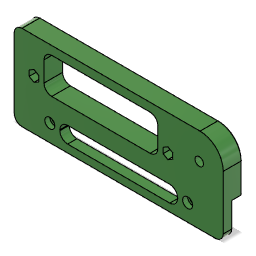
RFVplotter-PSUMountingBracketRight-v1_0 (Autodesk Fusion 360 design; units mm, degrees)
Autodesk Fusion 360 part; units mm, degrees
sketch "Sketch1" plane through (0, 0, 0) normal (0, 0, 1) x (1, 0, 0)
  line L0 (67.5, 27.5) -> (-67.5, 27.5)
  line L1 (-67.5, 27.5) -> (-67.5, -27.5)
  line L2 (-67.5, -27.5) -> (67.5, -27.5)
  line L3 (67.5, -27.5) -> (67.5, 27.5)
  line L4 (67.5, 27.5) -> (-67.5, -27.5) construction
  line L5 (-67.5, 27.5) -> (67.5, -27.5) construction
  dimension "d1" = 55
  dimension "d2" = 135
  constraint horizontal L0
  constraint perpendicular L0 L1
  constraint parallel L0 L2
  constraint parallel L1 L3
  constraint coincident L4 origin
  constraint coincident L5 origin
  measures "d1" distance of L0.end L1.end
  measures "d2" distance of L1.end L2.end
extrude "Extrude1" add sketch "Sketch1" along normal blind 6
sketch "Sketch3" plane through (0, 0, 0) normal (0, 0, -1) x (-1, 0, 0)
  line L0 (-67.5, 27.5) -> (-67.5, -27.5)
  line L1 (-67.5, -27.5) -> (67.5, -27.5)
  line L2 (67.5, -27.5) -> (67.5, 27.5)
  line L3 (67.5, 27.5) -> (-67.5, 27.5)
  line L4 (-67.5, -7) -> (67.5, -7)
  line L5 (67.5, -7) -> (67.5, 27.5)
  line L6 (67.5, 27.5) -> (-67.5, 27.5)
  line L7 (-67.5, 27.5) -> (-67.5, -7)
  line L8 (-67.5, -7) -> (67.5, 27.5) construction
  line L9 (67.5, -7) -> (-67.5, 27.5) construction
  point P0 (0, 10.25)
  dimension "d14" = 34.5
  dimension "d30" = 20.5
  constraint horizontal L4
  constraint perpendicular L4 L5
  constraint parallel L4 L6
  constraint parallel L5 L7
  constraint coincident L8 P0
  constraint coincident L9 P0
  constraint collinear L2 L5
  constraint collinear L3 L6
  constraint collinear L0 L7
  measures "d14" distance of L4.end L2.end
  measures "d30" distance of L1 L4
extrude "Extrude2" add sketch "Sketch3" along normal blind 6 contours L0 L2 L3 L4 L5 L6 L7
sketch "Sketch2" plane through (0, 0, 6) normal (0, 0, 1) x (1, 0, 0)
  line L0 (67.5, -27.5) -> (67.5, 27.5)
  line L1 (67.5, 27.5) -> (-67.5, 27.5)
  line L2 (-67.5, 27.5) -> (-67.5, -27.5)
  line L3 (-67.5, -27.5) -> (67.5, -27.5)
  line L4 (67.5, -7) -> (-67.5, -7)
  point P0 (-44.5, -16.5)
  point P1 (44.5, -16.5)
  dimension "d7" = 23
  dimension "d47" = 9.5
  dimension "d48" = 9.5
  dimension "d49" = 89
  measures "d7" distance of L0 P1
  measures "d47" distance of P1 L4
  measures "d48" distance of P0 L4
  measures "d49" horizontal distance of P0 P1
hole "Hole1" at (-44.5, -16.5, 6) at (44.5, -16.5, 6) direction (0, 0, -1) diameter 3.5 end through all counterbore diameter 6.5 counterbore depth 3.25
sketch "Sketch4" plane through (0, 0, -6) normal (0, 0, -1) x (-1, 0, 0)
  line L0 (-67.5, 27.5) -> (-67.5, -7)
  line L1 (-67.5, -7) -> (67.5, -7)
  line L2 (67.5, -7) -> (67.5, 27.5)
  line L3 (67.5, 27.5) -> (-67.5, 27.5)
  line L4 (-67.5, 4.75) -> (67.5, 4.75) construction
  point P0 (54.75, 4.75)
  point P1 (-31.75, 4.75)
  dimension "d19" = 12.75
  dimension "d20" = 86.5
  dimension "d31" = 11.75
  constraint coincident L0 L4.start
  constraint coincident L2 L4.end
  constraint perpendicular L2 L4
  constraint coincident L4 P0
  constraint coincident L4 P1
  measures "d19" distance of L2 P0
  measures "d20" distance of P0 P1
  measures "d31" distance of L1 L4
hole "Hole2" at (31.75, 4.75, -6) at (-54.75, 4.75, -6) direction (0, 0, 1) diameter 3.5 end through all
sketch "Sketch5" plane through (0, 0, 6) normal (0, 0, 1) x (1, 0, 0)
  circle A0 centre (31.75, 4.75) radius 1.75
  circle A1 centre (-54.75, 4.75) radius 1.75
  circle A2 centre (-44.5, -16.5) radius 3.25
  circle A3 centre (44.5, -16.5) radius 3.25
  line L0 (67.5, -27.5) -> (67.5, 27.5)
  line L1 (67.5, 27.5) -> (-67.5, 27.5)
  line L2 (-67.5, 27.5) -> (-67.5, -27.5)
  line L3 (-67.5, -27.5) -> (67.5, -27.5)
  line L4 (-51.65, 6.5398) -> (-54.75, 8.3296)
  line L5 (-54.75, 8.3296) -> (-57.85, 6.5398)
  line L6 (-57.85, 6.5398) -> (-57.85, 2.9602)
  line L7 (-57.85, 2.9602) -> (-54.75, 1.1704)
  line L8 (-54.75, 1.1704) -> (-51.65, 2.9602)
  line L9 (-51.65, 2.9602) -> (-51.65, 6.5398)
  line L10 (34.85, 2.9602) -> (34.85, 6.5398)
  line L11 (34.85, 6.5398) -> (31.75, 8.3296)
  line L12 (31.75, 8.3296) -> (28.65, 6.5398)
  line L13 (28.65, 6.5398) -> (28.65, 2.9602)
  line L14 (28.65, 2.9602) -> (31.75, 1.1704)
  line L15 (31.75, 1.1704) -> (34.85, 2.9602)
  point P0 (-54.75, 4.75)
  point P1 (31.75, 4.75)
  dimension "d24" = 6.2
  dimension "d25" = 6.2
  constraint coincident P0 A1.centre
  constraint vertical L9
  constraint coincident A0.centre P1
  constraint vertical L10
  measures "d24" distance of L6 L9
  measures "d25" distance of L10 L13
extrude "Extrude3" cut sketch "Sketch5" against normal blind 6 contours L4 L5 L6 L7 L8 L9 | L10 L11 L12 L13 L14 L15
sketch "Sketch6" plane through (0, 0, -6) normal (0, 0, -1) x (-1, 0, 0)
  circle A0 centre (-31.75, 4.75) radius 1.75
  circle A1 centre (54.75, 4.75) radius 1.75
  line L0 (-67.5, 27.5) -> (-67.5, -7)
  line L1 (-67.5, -7) -> (67.5, -7)
  line L2 (67.5, -7) -> (67.5, 27.5)
  line L3 (67.5, 27.5) -> (-67.5, 27.5)
  line L4 (59.5, -7) -> (-36.5, -7) construction
  line L5 (-36.5, -7) -> (-36.5, 28) construction
  line L6 (-36.5, 28) -> (59.5, 28) construction
  line L7 (59.5, 28) -> (59.5, -7) construction
  line L8 (59.5, -7) -> (-36.5, 28) construction
  line L9 (-36.5, -7) -> (59.5, 28) construction
  line L10 (11.5, 50.5144) -> (11.5, -41.0982) construction
  line L11 (-52, 27.5) -> (-52, -7) construction
  line L12 (-36.5, 10.25) -> (-67.5, 10.25) construction
  point P0 (11.5, 10.5)
  point P1 (-52, 10.25)
  dimension "d28" = 35
  dimension "d29" = 96
  constraint horizontal L4
  constraint perpendicular L4 L5
  constraint parallel L4 L6
  constraint parallel L5 L7
  constraint coincident L8 P0
  constraint coincident L9 P0
  constraint collinear L1 L4
  constraint perpendicular L4 L10
  constraint symmetric A0.centre A1.centre L10
  constraint coincident P0 L10
  constraint coincident L3 L11.start
  constraint coincident L1 L11.end
  constraint perpendicular L1 L11
  constraint coincident L5 L12.start
  constraint coincident L0 L12.end
  constraint perpendicular L0 L12
  constraint symmetric L1 L3 L12
  constraint coincident L11 P1
  constraint coincident L12 P1
  measures "d28" distance of L4.start L6.end
  measures "d29" distance of L5.end L6.end
hole "Hole3" at (52, 10.25, -6) direction (0, 0, 1) diameter 5.5 end through all
fillet "Fillet1" radius 5 2 edges at (67.5, -27.5, 3) (-67.5, -27.5, 3)
fillet "Fillet1" radius 5 1 edges at (-67.5, 27.5, 0)
fillet "Fillet3" radius 15 1 edges at (67.5, 27.5, 0)
fillet "Fillet4" radius 1 1 edges at (0, -7, -6)
fillet "Fillet5" radius 0.5 14 edges at (-67.5, -14.75, 0) (-66.0355, -26.0355, 0) (0, -27.5, 0) (66.0355, -26.0355, 0) (67.5, -14.75, 0) (-67.5, -7, -2.5) (-67.5, -6.7071, -5.7071) (-67.5, 8.25, -6) (-66.0355, 26.0355, -6) (-5, 27.5, -6) (63.1066, 23.1066, -6) (67.5, 3.25, -6) (67.5, -6.7071, -5.7071) (67.5, -7, -2.5)
sketch "Sketch7" plane through (0, 0, -6) normal (0, 0, -1) x (-1, 0, 0)
  line L0 (-67, 12.5) -> (-67, -6)
  line L1 (-67, -6) -> (67, -6)
  line L2 (67, -6) -> (67, 22.5)
  arc A0 (67, 22.5) -> (62.5, 27) centre (62.5, 22.5) ccw
  line L3 (62.5, 27) -> (-52.5, 27)
  arc A1 (-52.5, 27) -> (-67, 12.5) centre (-52.5, 12.5) ccw
  circle A2 centre (54.75, 4.75) radius 1.75
  circle A3 centre (-31.75, 4.75) radius 1.75
  circle A4 centre (-52, 10.25) radius 2.75
  line L4 (-25.25, 22) -> (48.25, 22)
  line L5 (48.25, 22) -> (48.25, -1)
  line L6 (48.25, -1) -> (-25.25, -1)
  line L7 (-25.25, -1) -> (-25.25, 22)
  line L8 (-25.25, 22) -> (48.25, -1) construction
  line L9 (48.25, 22) -> (-25.25, -1) construction
  point P0 (11.5, 10.5)
  dimension "d50" = 5
  dimension "d51" = 5
  dimension "d52" = 6.5
  dimension "d53" = 6.5
  constraint horizontal L4
  constraint perpendicular L4 L5
  constraint parallel L4 L6
  constraint parallel L5 L7
  constraint coincident L8 P0
  constraint coincident L9 P0
  measures "d50" distance of L3 L4
  measures "d51" distance of L1 L6
  measures "d52" distance of A2.centre L5
  measures "d53" distance of A3.centre L7
extrude "Extrude4" cut sketch "Sketch7" against normal through all contours L4 L5 L6 L7
fillet "Fillet6" radius 5 4 edges at (25.25, 22, 0) (25.25, -1, 0) (-48.25, -1, 0) (-48.25, 22, 0)
sketch "Sketch8" plane through (0, 0, 0) normal (0, 0, -1) x (-1, 0, 0)
  line L0 (-67, -7) -> (-67, -22.5)
  arc A0 (-67, -22.5) -> (-62.5, -27) centre (-62.5, -22.5) ccw
  line L1 (-62.5, -27) -> (62.5, -27)
  arc A1 (62.5, -27) -> (67, -22.5) centre (62.5, -22.5) ccw
  line L2 (67, -22.5) -> (67, -7)
  line L3 (67, -7) -> (-67, -7)
  circle A2 centre (-44.5, -16.5) radius 1.75
  circle A3 centre (44.5, -16.5) radius 1.75
  line L4 (38, -22.5) -> (-38, -22.5)
  line L5 (-38, -22.5) -> (-38, -12)
  line L6 (-38, -12) -> (38, -12)
  line L7 (38, -12) -> (38, -22.5)
  line L8 (38, -22.5) -> (-38, -12) construction
  line L9 (-38, -22.5) -> (38, -12) construction
  line L10 (-62.5, -27.5) -> (62.5, -27.5)
  point P0 (0, -17.25)
  dimension "d57" = 5
  dimension "d58" = 5
  dimension "d59" = 6.5
  dimension "d60" = 6.5
  constraint horizontal L4
  constraint perpendicular L4 L5
  constraint parallel L4 L6
  constraint parallel L5 L7
  constraint coincident L8 P0
  constraint coincident L9 P0
  measures "d57" distance of L3 L6
  measures "d58" distance of L4 L10
  measures "d59" distance of A2.centre L5
  measures "d60" distance of A3.centre L7
extrude "Extrude5" cut sketch "Sketch8" against normal through all contours L4 L5 L6 L7
fillet "Fillet7" radius 5 4 edges at (38, -12, 3) (38, -22.5, 3) (-38, -22.5, 3) (-38, -12, 3)
equation "d7 = 21.5 mm + 1.5 mm"
equation "d19 = 15 mm - 2.25 mm"
equation "d20 = 82 mm + 4.5 mm"
equation "d25 = d24"
equation "d31 = 9.5 mm + 2.25 mm"
equation "d51 = d50"
equation "d53 = d52"
equation "d58 = d57"
equation "d60 = d59"
